Autodesk Fusion 360 part; units mm, degrees
note: some values were not read from the file. Chosen so that the rebuilt part matches the saved one: which bodies a step acts on.
(part 3 of 3)
  arc A266 (-250.9457, 90.0604) -> (-250.4457, 89.5604) centre (-250.4457, 90.0604) ccw
  line L293 (-250.9457, 90.0604) -> (-250.9457, 90.3732)
  line L294 (-250.9457, 90.3732) -> (-252.5563, 90.3732)
  line L295 (-252.5563, 90.3732) -> (-252.5563, 88.75)
  arc A267 (-253.0563, 88.25) -> (-252.5563, 88.75) centre (-253.0563, 88.75) ccw
  line L296 (-253.0563, 88.25) -> (-266.0562, 88.25)
  arc A268 (-266.5562, 88.75) -> (-266.0563, 88.25) centre (-266.0563, 88.75) ccw
  line L297 (-266.5562, 88.75) -> (-266.5562, 90.3732)
  line L298 (-266.5562, 90.3732) -> (-268.1669, 90.3732)
  line L299 (-268.1669, 90.3732) -> (-268.1669, 90.0604)
  arc A269 (-268.6669, 89.5604) -> (-268.1669, 90.0604) centre (-268.6669, 90.0604) ccw
  line L300 (-268.6669, 89.5604) -> (-274.3216, 89.5604)
  arc A270 (-274.8216, 90.0604) -> (-274.3216, 89.5604) centre (-274.3216, 90.0604) ccw
  line L301 (-274.8216, 90.0604) -> (-274.8216, 92.964)
  line L302 (-274.8216, 92.964) -> (-275.1852, 92.964)
  arc A271 (-275.6852, 93.464) -> (-275.1852, 92.964) centre (-275.1852, 93.464) ccw
  line L303 (-275.6852, 93.464) -> (-275.6852, 95.758)
  arc A272 (-83.9875, 88.25) -> (-83.4875, 88.75) centre (-83.9875, 88.75) ccw
  line L304 (-83.9875, 88.25) -> (-96.9875, 88.25)
  arc A273 (-97.4875, 88.75) -> (-96.9875, 88.25) centre (-96.9875, 88.75) ccw
  line L305 (-97.4875, 88.75) -> (-97.4875, 101.75)
  arc A274 (-96.9875, 102.25) -> (-97.4875, 101.75) centre (-96.9875, 101.75) ccw
  line L306 (-96.9875, 102.25) -> (-83.9875, 102.25)
  arc A275 (-83.4875, 101.75) -> (-83.9875, 102.25) centre (-83.9875, 101.75) ccw
  line L307 (-83.4875, 101.75) -> (-83.4875, 88.75)
  arc A276 (-112.5625, 69.2) -> (-112.0625, 69.7) centre (-112.5625, 69.7) ccw
  line L308 (-112.5625, 69.2) -> (-125.5625, 69.2)
  arc A277 (-126.0625, 69.7) -> (-125.5625, 69.2) centre (-125.5625, 69.7) ccw
  line L309 (-126.0625, 69.7) -> (-126.0625, 82.7)
  arc A278 (-125.5625, 83.2) -> (-126.0625, 82.7) centre (-125.5625, 82.7) ccw
  line L310 (-125.5625, 83.2) -> (-112.5625, 83.2)
  arc A279 (-112.0625, 82.7) -> (-112.5625, 83.2) centre (-112.5625, 82.7) ccw
  line L311 (-112.0625, 82.7) -> (-112.0625, 69.7)
  arc A280 (-198.2875, 88.25) -> (-197.7875, 88.75) centre (-198.2875, 88.75) ccw
  line L312 (-198.2875, 88.25) -> (-211.2875, 88.25)
  arc A281 (-211.7875, 88.75) -> (-211.2875, 88.25) centre (-211.2875, 88.75) ccw
  line L313 (-211.7875, 88.75) -> (-211.7875, 101.75)
  arc A282 (-211.2875, 102.25) -> (-211.7875, 101.75) centre (-211.2875, 101.75) ccw
  line L314 (-211.2875, 102.25) -> (-198.2875, 102.25)
  arc A283 (-197.7875, 101.75) -> (-198.2875, 102.25) centre (-198.2875, 101.75) ccw
  line L315 (-197.7875, 101.75) -> (-197.7875, 88.75)
  arc A284 (-207.8125, 69.2) -> (-207.3125, 69.7) centre (-207.8125, 69.7) ccw
  line L316 (-207.8125, 69.2) -> (-220.8125, 69.2)
  arc A285 (-221.3125, 69.7) -> (-220.8125, 69.2) centre (-220.8125, 69.7) ccw
  line L317 (-221.3125, 69.7) -> (-221.3125, 82.7)
  arc A286 (-220.8125, 83.2) -> (-221.3125, 82.7) centre (-220.8125, 82.7) ccw
  line L318 (-220.8125, 83.2) -> (-207.8125, 83.2)
  arc A287 (-207.3125, 82.7) -> (-207.8125, 83.2) centre (-207.8125, 82.7) ccw
  line L319 (-207.3125, 82.7) -> (-207.3125, 69.7)
  arc A288 (-45.8875, 88.25) -> (-45.3875, 88.75) centre (-45.8875, 88.75) ccw
  line L320 (-45.8875, 88.25) -> (-58.8875, 88.25)
  arc A289 (-59.3875, 88.75) -> (-58.8875, 88.25) centre (-58.8875, 88.75) ccw
  line L321 (-59.3875, 88.75) -> (-59.3875, 101.75)
  arc A290 (-58.8875, 102.25) -> (-59.3875, 101.75) centre (-58.8875, 101.75) ccw
  line L322 (-58.8875, 102.25) -> (-45.8875, 102.25)
  arc A291 (-45.3875, 101.75) -> (-45.8875, 102.25) centre (-45.8875, 101.75) ccw
  line L323 (-45.3875, 101.75) -> (-45.3875, 88.75)
  arc A292 (-122.0875, 88.25) -> (-121.5875, 88.75) centre (-122.0875, 88.75) ccw
  line L324 (-122.0875, 88.25) -> (-135.0875, 88.25)
  arc A293 (-135.5875, 88.75) -> (-135.0875, 88.25) centre (-135.0875, 88.75) ccw
  line L325 (-135.5875, 88.75) -> (-135.5875, 101.75)
  arc A294 (-135.0875, 102.25) -> (-135.5875, 101.75) centre (-135.0875, 101.75) ccw
  line L326 (-135.0875, 102.25) -> (-122.0875, 102.25)
  arc A295 (-121.5875, 101.75) -> (-122.0875, 102.25) centre (-122.0875, 101.75) ccw
  line L327 (-121.5875, 101.75) -> (-121.5875, 88.75)
  arc A296 (-179.2375, 88.25) -> (-178.7375, 88.75) centre (-179.2375, 88.75) ccw
  line L328 (-179.2375, 88.25) -> (-192.2375, 88.25)
  arc A297 (-192.7375, 88.75) -> (-192.2375, 88.25) centre (-192.2375, 88.75) ccw
  line L329 (-192.7375, 88.75) -> (-192.7375, 101.75)
  arc A298 (-192.2375, 102.25) -> (-192.7375, 101.75) centre (-192.2375, 101.75) ccw
  line L330 (-192.2375, 102.25) -> (-179.2375, 102.25)
  arc A299 (-178.7375, 101.75) -> (-179.2375, 102.25) centre (-179.2375, 101.75) ccw
  line L331 (-178.7375, 101.75) -> (-178.7375, 88.75)
  arc A300 (-136.375, 31.1) -> (-135.875, 31.6) centre (-136.375, 31.6) ccw
  line L332 (-136.375, 31.1) -> (-149.375, 31.1)
  arc A301 (-149.875, 31.6) -> (-149.375, 31.1) centre (-149.375, 31.6) ccw
  line L333 (-149.875, 31.6) -> (-149.875, 44.6)
  arc A302 (-149.375, 45.1) -> (-149.875, 44.6) centre (-149.375, 44.6) ccw
  line L334 (-149.375, 45.1) -> (-136.375, 45.1)
  arc A303 (-135.875, 44.6) -> (-136.375, 45.1) centre (-136.375, 44.6) ccw
  line L335 (-135.875, 44.6) -> (-135.875, 31.6)
  arc A304 (-93.5125, 69.2) -> (-93.0125, 69.7) centre (-93.5125, 69.7) ccw
  line L336 (-93.5125, 69.2) -> (-106.5125, 69.2)
  arc A305 (-107.0125, 69.7) -> (-106.5125, 69.2) centre (-106.5125, 69.7) ccw
  line L337 (-107.0125, 69.7) -> (-107.0125, 82.7)
  arc A306 (-106.5125, 83.2) -> (-107.0125, 82.7) centre (-106.5125, 82.7) ccw
  line L338 (-106.5125, 83.2) -> (-93.5125, 83.2)
  arc A307 (-93.0125, 82.7) -> (-93.5125, 83.2) centre (-93.5125, 82.7) ccw
  line L339 (-93.0125, 82.7) -> (-93.0125, 69.7)
  arc A308 (-31.6, 50.15) -> (-31.1, 50.65) centre (-31.6, 50.65) ccw
  line L340 (-31.6, 50.15) -> (-44.6, 50.15)
  arc A309 (-45.1, 50.65) -> (-44.6, 50.15) centre (-44.6, 50.65) ccw
  line L341 (-45.1, 50.65) -> (-45.1, 63.65)
  arc A310 (-44.6, 64.15) -> (-45.1, 63.65) centre (-44.6, 63.65) ccw
  line L342 (-44.6, 64.15) -> (-31.6, 64.15)
  arc A311 (-31.1, 63.65) -> (-31.6, 64.15) centre (-31.6, 63.65) ccw
  line L343 (-31.1, 63.65) -> (-31.1, 50.65)
  line L344 (-282.829, 38.608) -> (-282.4654, 38.608)
  arc A312 (-282.4654, 38.608) -> (-281.9654, 39.108) centre (-282.4654, 39.108) ccw
  line L345 (-281.9654, 39.108) -> (-281.9654, 44.204)
  arc A313 (-281.4654, 44.704) -> (-281.9654, 44.204) centre (-281.4654, 44.204) ccw
  line L346 (-281.4654, 44.704) -> (-280.662, 44.704)
  arc A314 (-280.662, 44.704) -> (-280.162, 45.204) centre (-280.662, 45.204) ccw
  line L347 (-280.162, 45.204) -> (-280.162, 45.3724)
  arc A315 (-279.662, 45.8724) -> (-280.162, 45.3724) centre (-279.662, 45.3724) ccw
  line L348 (-279.662, 45.8724) -> (-277.614, 45.8724)
  arc A316 (-277.114, 45.3724) -> (-277.614, 45.8724) centre (-277.614, 45.3724) ccw
  line L349 (-277.114, 45.3724) -> (-277.114, 45.204)
  arc A317 (-277.114, 45.204) -> (-276.614, 44.704) centre (-276.614, 45.204) ccw
  line L350 (-276.614, 44.704) -> (-275.3106, 44.704)
  line L351 (-275.3106, 44.704) -> (-275.3106, 44.4166)
  arc A318 (-275.3106, 44.4166) -> (-274.8106, 43.9166) centre (-274.8106, 44.4166) ccw
  line L352 (-274.8106, 43.9166) -> (-273.7, 43.9166)
  line L353 (-273.7, 43.9166) -> (-273.7, 44.6)
  arc A319 (-273.2, 45.1) -> (-273.7, 44.6) centre (-273.2, 44.6) ccw
  line L354 (-273.2, 45.1) -> (-260.2, 45.1)
  arc A320 (-259.7, 44.6) -> (-260.2, 45.1) centre (-260.2, 44.6) ccw
  line L355 (-259.7, 44.6) -> (-259.7, 43.9166)
  line L356 (-259.7, 43.9166) -> (-258.5894, 43.9166)
  arc A321 (-258.5894, 43.9166) -> (-258.0894, 44.4166) centre (-258.5894, 44.4166) ccw
  line L357 (-258.0894, 44.4166) -> (-258.0894, 44.704)
  line L358 (-258.0894, 44.704) -> (-256.786, 44.704)
  arc A322 (-256.786, 44.704) -> (-256.286, 45.204) centre (-256.786, 45.204) ccw
  line L359 (-256.286, 45.204) -> (-256.286, 45.3724)
  arc A323 (-255.786, 45.8724) -> (-256.286, 45.3724) centre (-255.786, 45.3724) ccw
  line L360 (-255.786, 45.8724) -> (-253.738, 45.8724)
  arc A324 (-253.238, 45.3724) -> (-253.738, 45.8724) centre (-253.738, 45.3724) ccw
  line L361 (-253.238, 45.3724) -> (-253.238, 45.204)
  arc A325 (-253.238, 45.204) -> (-252.738, 44.704) centre (-252.738, 45.204) ccw
  line L362 (-252.738, 44.704) -> (-251.9346, 44.704)
  arc A326 (-251.4346, 44.204) -> (-251.9346, 44.704) centre (-251.9346, 44.204) ccw
  line L363 (-251.4346, 44.204) -> (-251.4346, 39.108)
  arc A327 (-251.4346, 39.108) -> (-250.9346, 38.608) centre (-250.9346, 39.108) ccw
  line L364 (-250.9346, 38.608) -> (-250.571, 38.608)
  line L365 (-250.571, 38.608) -> (-250.571, 36.314)
  arc A328 (-251.071, 35.814) -> (-250.571, 36.314) centre (-251.071, 36.314) ccw
  line L366 (-251.071, 35.814) -> (-251.4346, 35.814)
  line L367 (-251.4346, 35.814) -> (-251.4346, 32.9104)
  arc A329 (-251.9346, 32.4104) -> (-251.4346, 32.9104) centre (-251.9346, 32.9104) ccw
  line L368 (-251.9346, 32.4104) -> (-257.5894, 32.4104)
  arc A330 (-258.0894, 32.9104) -> (-257.5894, 32.4104) centre (-257.5894, 32.9104) ccw
  line L369 (-258.0894, 32.9104) -> (-258.0894, 33.2232)
  line L370 (-258.0894, 33.2232) -> (-259.7, 33.2232)
  line L371 (-259.7, 33.2232) -> (-259.7, 31.6)
  arc A331 (-260.2, 31.1) -> (-259.7, 31.6) centre (-260.2, 31.6) ccw
  line L372 (-260.2, 31.1) -> (-273.2, 31.1)
  arc A332 (-273.7, 31.6) -> (-273.2, 31.1) centre (-273.2, 31.6) ccw
  line L373 (-273.7, 31.6) -> (-273.7, 33.2232)
  line L374 (-273.7, 33.2232) -> (-275.3106, 33.2232)
  line L375 (-275.3106, 33.2232) -> (-275.3106, 32.9104)
  arc A333 (-275.8106, 32.4104) -> (-275.3106, 32.9104) centre (-275.8106, 32.9104) ccw
  line L376 (-275.8106, 32.4104) -> (-281.4654, 32.4104)
  arc A334 (-281.9654, 32.9104) -> (-281.4654, 32.4104) centre (-281.4654, 32.9104) ccw
  line L377 (-281.9654, 32.9104) -> (-281.9654, 35.814)
  line L378 (-281.9654, 35.814) -> (-282.329, 35.814)
  arc A335 (-282.829, 36.314) -> (-282.329, 35.814) centre (-282.329, 36.314) ccw
  line L379 (-282.829, 36.314) -> (-282.829, 38.608)
  arc A336 (-50.65, 50.15) -> (-50.15, 50.65) centre (-50.65, 50.65) ccw
  line L380 (-50.65, 50.15) -> (-63.65, 50.15)
  arc A337 (-64.15, 50.65) -> (-63.65, 50.15) centre (-63.65, 50.65) ccw
  line L381 (-64.15, 50.65) -> (-64.15, 63.65)
  arc A338 (-63.65, 64.15) -> (-64.15, 63.65) centre (-63.65, 63.65) ccw
  line L382 (-63.65, 64.15) -> (-50.65, 64.15)
  arc A339 (-50.15, 63.65) -> (-50.65, 64.15) centre (-50.65, 63.65) ccw
  line L383 (-50.15, 63.65) -> (-50.15, 50.65)
  arc A340 (-3.025, 2.525) -> (-2.525, 3.025) centre (-3.025, 3.025) ccw
  line L384 (-3.025, 2.525) -> (-16.025, 2.525)
  arc A341 (-16.525, 3.025) -> (-16.025, 2.525) centre (-16.025, 3.025) ccw
  line L385 (-16.525, 3.025) -> (-16.525, 16.025)
  arc A342 (-16.025, 16.525) -> (-16.525, 16.025) centre (-16.025, 16.025) ccw
  line L386 (-16.025, 16.525) -> (-3.025, 16.525)
  arc A343 (-2.525, 16.025) -> (-3.025, 16.525) centre (-3.025, 16.025) ccw
  line L387 (-2.525, 16.025) -> (-2.525, 3.025)
  arc A344 (-88.75, 50.15) -> (-88.25, 50.65) centre (-88.75, 50.65) ccw
  line L388 (-88.75, 50.15) -> (-101.75, 50.15)
  arc A345 (-102.25, 50.65) -> (-101.75, 50.15) centre (-101.75, 50.65) ccw
  line L389 (-102.25, 50.65) -> (-102.25, 63.65)
  arc A346 (-101.75, 64.15) -> (-102.25, 63.65) centre (-101.75, 63.65) ccw
  line L390 (-101.75, 64.15) -> (-88.75, 64.15)
  arc A347 (-88.25, 63.65) -> (-88.75, 64.15) centre (-88.75, 63.65) ccw
  line L391 (-88.25, 63.65) -> (-88.25, 50.65)
  arc A348 (-145.9, 50.15) -> (-145.4, 50.65) centre (-145.9, 50.65) ccw
  line L392 (-145.9, 50.15) -> (-158.9, 50.15)
  arc A349 (-159.4, 50.65) -> (-158.9, 50.15) centre (-158.9, 50.65) ccw
  line L393 (-159.4, 50.65) -> (-159.4, 63.65)
  arc A350 (-158.9, 64.15) -> (-159.4, 63.65) centre (-158.9, 63.65) ccw
  line L394 (-158.9, 64.15) -> (-145.9, 64.15)
  arc A351 (-145.4, 63.65) -> (-145.9, 64.15) centre (-145.9, 63.65) ccw
  line L395 (-145.4, 63.65) -> (-145.4, 50.65)
  arc A352 (-60.175, 2.525) -> (-59.675, 3.025) centre (-60.175, 3.025) ccw
  line L396 (-60.175, 2.525) -> (-73.175, 2.525)
  arc A353 (-73.675, 3.025) -> (-73.175, 2.525) centre (-73.175, 3.025) ccw
  line L397 (-73.675, 3.025) -> (-73.675, 16.025)
  arc A354 (-73.175, 16.525) -> (-73.675, 16.025) centre (-73.175, 16.025) ccw
  line L398 (-73.175, 16.525) -> (-60.175, 16.525)
  arc A355 (-59.675, 16.025) -> (-60.175, 16.525) centre (-60.175, 16.025) ccw
  line L399 (-59.675, 16.025) -> (-59.675, 3.025)
  arc A356 (-293.5375, 31.1) -> (-293.0375, 31.6) centre (-293.5375, 31.6) ccw
  line L400 (-293.5375, 31.1) -> (-306.5375, 31.1)
  arc A357 (-307.0375, 31.6) -> (-306.5375, 31.1) centre (-306.5375, 31.6) ccw
  line L401 (-307.0375, 31.6) -> (-307.0375, 44.6)
  arc A358 (-306.5375, 45.1) -> (-307.0375, 44.6) centre (-306.5375, 44.6) ccw
  line L402 (-306.5375, 45.1) -> (-293.5375, 45.1)
  arc A359 (-293.0375, 44.6) -> (-293.5375, 45.1) centre (-293.5375, 44.6) ccw
  line L403 (-293.0375, 44.6) -> (-293.0375, 31.6)
  arc A360 (-312.5875, 2.525) -> (-312.0875, 3.025) centre (-312.5875, 3.025) ccw
  line L404 (-312.5875, 2.525) -> (-325.5875, 2.525)
  arc A361 (-326.0875, 3.025) -> (-325.5875, 2.525) centre (-325.5875, 3.025) ccw
  line L405 (-326.0875, 3.025) -> (-326.0875, 16.025)
  arc A362 (-325.5875, 16.525) -> (-326.0875, 16.025) centre (-325.5875, 16.025) ccw
  line L406 (-325.5875, 16.525) -> (-312.5875, 16.525)
  arc A363 (-312.0875, 16.025) -> (-312.5875, 16.525) centre (-312.5875, 16.025) ccw
  line L407 (-312.0875, 16.025) -> (-312.0875, 3.025)
  arc A364 (-164.95, 50.15) -> (-164.45, 50.65) centre (-164.95, 50.65) ccw
  line L408 (-164.95, 50.15) -> (-177.95, 50.15)
  arc A365 (-178.45, 50.65) -> (-177.95, 50.15) centre (-177.95, 50.65) ccw
  line L409 (-178.45, 50.65) -> (-178.45, 63.65)
  arc A366 (-177.95, 64.15) -> (-178.45, 63.65) centre (-177.95, 63.65) ccw
  line L410 (-177.95, 64.15) -> (-164.95, 64.15)
  arc A367 (-164.45, 63.65) -> (-164.95, 64.15) centre (-164.95, 63.65) ccw
  line L411 (-164.45, 63.65) -> (-164.45, 50.65)
  arc A368 (-107.8, 50.15) -> (-107.3, 50.65) centre (-107.8, 50.65) ccw
  line L412 (-107.8, 50.15) -> (-120.8, 50.15)
  arc A369 (-121.3, 50.65) -> (-120.8, 50.15) centre (-120.8, 50.65) ccw
  line L413 (-121.3, 50.65) -> (-121.3, 63.65)
  arc A370 (-120.8, 64.15) -> (-121.3, 63.65) centre (-120.8, 63.65) ccw
  line L414 (-120.8, 64.15) -> (-107.8, 64.15)
  arc A371 (-107.3, 63.65) -> (-107.8, 64.15) centre (-107.8, 63.65) ccw
  line L415 (-107.3, 63.65) -> (-107.3, 50.65)
  arc A372 (-150.6625, 69.2) -> (-150.1625, 69.7) centre (-150.6625, 69.7) ccw
  line L416 (-150.6625, 69.2) -> (-163.6625, 69.2)
  arc A373 (-164.1625, 69.7) -> (-163.6625, 69.2) centre (-163.6625, 69.7) ccw
  line L417 (-164.1625, 69.7) -> (-164.1625, 82.7)
  arc A374 (-163.6625, 83.2) -> (-164.1625, 82.7) centre (-163.6625, 82.7) ccw
  line L418 (-163.6625, 83.2) -> (-150.6625, 83.2)
  arc A375 (-150.1625, 82.7) -> (-150.6625, 83.2) centre (-150.6625, 82.7) ccw
  line L419 (-150.1625, 82.7) -> (-150.1625, 69.7)
  arc A376 (-174.475, 31.1) -> (-173.975, 31.6) centre (-174.475, 31.6) ccw
  line L420 (-174.475, 31.1) -> (-187.475, 31.1)
  arc A377 (-187.975, 31.6) -> (-187.475, 31.1) centre (-187.475, 31.6) ccw
  line L421 (-187.975, 31.6) -> (-187.975, 44.6)
  arc A378 (-187.475, 45.1) -> (-187.975, 44.6) centre (-187.475, 44.6) ccw
  line L422 (-187.475, 45.1) -> (-174.475, 45.1)
  arc A379 (-173.975, 44.6) -> (-174.475, 45.1) centre (-174.475, 44.6) ccw
  line L423 (-173.975, 44.6) -> (-173.975, 31.6)
  arc A380 (-241.15, 50.15) -> (-240.65, 50.65) centre (-241.15, 50.65) ccw
  line L424 (-241.15, 50.15) -> (-254.15, 50.15)
  arc A381 (-254.65, 50.65) -> (-254.15, 50.15) centre (-254.15, 50.65) ccw
  line L425 (-254.65, 50.65) -> (-254.65, 63.65)
  arc A382 (-254.15, 64.15) -> (-254.65, 63.65) centre (-254.15, 63.65) ccw
  line L426 (-254.15, 64.15) -> (-241.15, 64.15)
  arc A383 (-240.65, 63.65) -> (-241.15, 64.15) centre (-241.15, 63.65) ccw
  line L427 (-240.65, 63.65) -> (-240.65, 50.65)
  arc A384 (-5.4063, 88.25) -> (-4.9063, 88.75) centre (-5.4062, 88.75) ccw
  line L428 (-5.4062, 88.25) -> (-18.4062, 88.25)
  arc A385 (-18.9062, 88.75) -> (-18.4062, 88.25) centre (-18.4062, 88.75) ccw
  line L429 (-18.9062, 88.75) -> (-18.9062, 101.75)
  arc A386 (-18.4062, 102.25) -> (-18.9063, 101.75) centre (-18.4063, 101.75) ccw
  line L430 (-18.4062, 102.25) -> (-5.4062, 102.25)
  arc A387 (-4.9062, 101.75) -> (-5.4062, 102.25) centre (-5.4062, 101.75) ccw
  line L431 (-4.9062, 101.75) -> (-4.9063, 88.75)
  arc A388 (-10.1687, 69.2) -> (-9.6687, 69.7) centre (-10.1687, 69.7) ccw
  line L432 (-10.1687, 69.2) -> (-23.1687, 69.2)
  arc A389 (-23.6687, 69.7) -> (-23.1687, 69.2) centre (-23.1688, 69.7) ccw
  line L433 (-23.6687, 69.7) -> (-23.6688, 82.7)
  arc A390 (-23.1687, 83.2) -> (-23.6687, 82.7) centre (-23.1688, 82.7) ccw
  line L434 (-23.1687, 83.2) -> (-10.1687, 83.2)
  arc A391 (-9.6687, 82.7) -> (-10.1687, 83.2) centre (-10.1688, 82.7) ccw
  line L435 (-9.6687, 82.7) -> (-9.6687, 69.7)
  arc A392 (-36.3625, 69.2) -> (-35.8625, 69.7) centre (-36.3625, 69.7) ccw
  line L436 (-36.3625, 69.2) -> (-49.3625, 69.2)
  arc A393 (-49.8625, 69.7) -> (-49.3625, 69.2) centre (-49.3625, 69.7) ccw
  line L437 (-49.8625, 69.7) -> (-49.8625, 82.7)
  arc A394 (-49.3625, 83.2) -> (-49.8625, 82.7) centre (-49.3625, 82.7) ccw
  line L438 (-49.3625, 83.2) -> (-36.3625, 83.2)
  arc A395 (-35.8625, 82.7) -> (-36.3625, 83.2) centre (-36.3625, 82.7) ccw
  line L439 (-35.8625, 82.7) -> (-35.8625, 69.7)
  arc A396 (-7.7875, 50.15) -> (-7.2875, 50.65) centre (-7.7875, 50.65) ccw
  line L440 (-7.7875, 50.15) -> (-20.7875, 50.15)
  arc A397 (-21.2875, 50.65) -> (-20.7875, 50.15) centre (-20.7875, 50.65) ccw
  line L441 (-21.2875, 50.65) -> (-21.2875, 63.65)
  arc A398 (-20.7875, 64.15) -> (-21.2875, 63.65) centre (-20.7875, 63.65) ccw
  line L442 (-20.7875, 64.15) -> (-7.7875, 64.15)
  arc A399 (-7.2875, 63.65) -> (-7.7875, 64.15) centre (-7.7875, 63.65) ccw
  line L443 (-7.2875, 63.65) -> (-7.2875, 50.65)
  arc A400 (-331.6375, 50.15) -> (-331.1375, 50.65) centre (-331.6375, 50.65) ccw
  line L444 (-331.6375, 50.15) -> (-344.6375, 50.15)
  arc A401 (-345.1375, 50.65) -> (-344.6375, 50.15) centre (-344.6375, 50.65) ccw
  line L445 (-345.1375, 50.65) -> (-345.1375, 63.65)
  arc A402 (-344.6375, 64.15) -> (-345.1375, 63.65) centre (-344.6375, 63.65) ccw
  line L446 (-344.6375, 64.15) -> (-331.6375, 64.15)
  arc A403 (-331.1375, 63.65) -> (-331.6375, 64.15) centre (-331.6375, 63.65) ccw
  line L447 (-331.1375, 63.65) -> (-331.1375, 50.65)
  arc A404 (-41.125, 2.525) -> (-40.625, 3.025) centre (-41.125, 3.025) ccw
  line L448 (-41.125, 2.525) -> (-54.125, 2.525)
  arc A405 (-54.625, 3.025) -> (-54.125, 2.525) centre (-54.125, 3.025) ccw
  line L449 (-54.625, 3.025) -> (-54.625, 16.025)
  arc A406 (-54.125, 16.525) -> (-54.625, 16.025) centre (-54.125, 16.025) ccw
  line L450 (-54.125, 16.525) -> (-41.125, 16.525)
  arc A407 (-40.625, 16.025) -> (-41.125, 16.525) centre (-41.125, 16.025) ccw
  line L451 (-40.625, 16.025) -> (-40.625, 3.025)
  arc A408 (-293.5375, 50.15) -> (-293.0375, 50.65) centre (-293.5375, 50.65) ccw
  line L452 (-293.5375, 50.15) -> (-306.5375, 50.15)
  arc A409 (-307.0375, 50.65) -> (-306.5375, 50.15) centre (-306.5375, 50.65) ccw
  line L453 (-307.0375, 50.65) -> (-307.0375, 63.65)
  arc A410 (-306.5375, 64.15) -> (-307.0375, 63.65) centre (-306.5375, 63.65) ccw
  line L454 (-306.5375, 64.15) -> (-293.5375, 64.15)
  arc A411 (-293.0375, 63.65) -> (-293.5375, 64.15) centre (-293.5375, 63.65) ccw
  line L455 (-293.0375, 63.65) -> (-293.0375, 50.65)
  arc A412 (-226.8625, 69.2) -> (-226.3625, 69.7) centre (-226.8625, 69.7) ccw
  line L456 (-226.8625, 69.2) -> (-239.8625, 69.2)
  arc A413 (-240.3625, 69.7) -> (-239.8625, 69.2) centre (-239.8625, 69.7) ccw
  line L457 (-240.3625, 69.7) -> (-240.3625, 82.7)
  arc A414 (-239.8625, 83.2) -> (-240.3625, 82.7) centre (-239.8625, 82.7) ccw
  line L458 (-239.8625, 83.2) -> (-226.8625, 83.2)
  arc A415 (-226.3625, 82.7) -> (-226.8625, 83.2) centre (-226.8625, 82.7) ccw
  line L459 (-226.3625, 82.7) -> (-226.3625, 69.7)
  arc A416 (-222.1, 50.15) -> (-221.6, 50.65) centre (-222.1, 50.65) ccw
  line L460 (-222.1, 50.15) -> (-235.1, 50.15)
  arc A417 (-235.6, 50.65) -> (-235.1, 50.15) centre (-235.1, 50.65) ccw
  line L461 (-235.6, 50.65) -> (-235.6, 63.65)
  arc A418 (-235.1, 64.15) -> (-235.6, 63.65) centre (-235.1, 63.65) ccw
  line L462 (-235.1, 64.15) -> (-222.1, 64.15)
  arc A419 (-221.6, 63.65) -> (-222.1, 64.15) centre (-222.1, 63.65) ccw
  line L463 (-221.6, 63.65) -> (-221.6, 50.65)
  arc A420 (-69.7, 50.15) -> (-69.2, 50.65) centre (-69.7, 50.65) ccw
  line L464 (-69.7, 50.15) -> (-82.7, 50.15)
  arc A421 (-83.2, 50.65) -> (-82.7, 50.15) centre (-82.7, 50.65) ccw
  line L465 (-83.2, 50.65) -> (-83.2, 63.65)
  arc A422 (-82.7, 64.15) -> (-83.2, 63.65) centre (-82.7, 63.65) ccw
  line L466 (-82.7, 64.15) -> (-69.7, 64.15)
  arc A423 (-69.2, 63.65) -> (-69.7, 64.15) centre (-69.7, 63.65) ccw
  line L467 (-69.2, 63.65) -> (-69.2, 50.65)
  arc A424 (-293.5375, 69.2) -> (-293.0375, 69.7) centre (-293.5375, 69.7) ccw
  line L468 (-293.5375, 69.2) -> (-306.5375, 69.2)
  arc A425 (-307.0375, 69.7) -> (-306.5375, 69.2) centre (-306.5375, 69.7) ccw
  line L469 (-307.0375, 69.7) -> (-307.0375, 82.7)
  arc A426 (-306.5375, 83.2) -> (-307.0375, 82.7) centre (-306.5375, 82.7) ccw
  line L470 (-306.5375, 83.2) -> (-293.5375, 83.2)
  arc A427 (-293.0375, 82.7) -> (-293.5375, 83.2) centre (-293.5375, 82.7) ccw
  line L471 (-293.0375, 82.7) -> (-293.0375, 69.7)
  arc A428 (-293.5375, 2.525) -> (-293.0375, 3.025) centre (-293.5375, 3.025) ccw
  line L472 (-293.5375, 2.525) -> (-306.5375, 2.525)
  arc A429 (-307.0375, 3.025) -> (-306.5375, 2.525) centre (-306.5375, 3.025) ccw
  line L473 (-307.0375, 3.025) -> (-307.0375, 16.025)
  arc A430 (-306.5375, 16.525) -> (-307.0375, 16.025) centre (-306.5375, 16.025) ccw
  line L474 (-306.5375, 16.525) -> (-293.5375, 16.525)
  arc A431 (-293.0375, 16.025) -> (-293.5375, 16.525) centre (-293.5375, 16.025) ccw
  line L475 (-293.0375, 16.025) -> (-293.0375, 3.025)
  arc A432 (-203.05, 50.15) -> (-202.55, 50.65) centre (-203.05, 50.65) ccw
  line L476 (-203.05, 50.15) -> (-216.05, 50.15)
  arc A433 (-216.55, 50.65) -> (-216.05, 50.15) centre (-216.05, 50.65) ccw
  line L477 (-216.55, 50.65) -> (-216.55, 63.65)
  arc A434 (-216.05, 64.15) -> (-216.55, 63.65) centre (-216.05, 63.65) ccw
  line L478 (-216.05, 64.15) -> (-203.05, 64.15)
  arc A435 (-202.55, 63.65) -> (-203.05, 64.15) centre (-203.05, 63.65) ccw
  line L479 (-202.55, 63.65) -> (-202.55, 50.65)
  arc A436 (-55.4125, 69.2) -> (-54.9125, 69.7) centre (-55.4125, 69.7) ccw
  line L480 (-55.4125, 69.2) -> (-68.4125, 69.2)
  arc A437 (-68.9125, 69.7) -> (-68.4125, 69.2) centre (-68.4125, 69.7) ccw
  line L481 (-68.9125, 69.7) -> (-68.9125, 82.7)
  arc A438 (-68.4125, 83.2) -> (-68.9125, 82.7) centre (-68.4125, 82.7) ccw
  line L482 (-68.4125, 83.2) -> (-55.4125, 83.2)
  arc A439 (-54.9125, 82.7) -> (-55.4125, 83.2) centre (-55.4125, 82.7) ccw
  line L483 (-54.9125, 82.7) -> (-54.9125, 69.7)
  arc A440 (-26.8375, 88.25) -> (-26.3375, 88.75) centre (-26.8375, 88.75) ccw
  line L484 (-26.8375, 88.25) -> (-39.8375, 88.25)
  arc A441 (-40.3375, 88.75) -> (-39.8375, 88.25) centre (-39.8375, 88.75) ccw
  line L485 (-40.3375, 88.75) -> (-40.3375, 101.75)
  arc A442 (-39.8375, 102.25) -> (-40.3375, 101.75) centre (-39.8375, 101.75) ccw
  line L486 (-39.8375, 102.25) -> (-26.8375, 102.25)
  arc A443 (-26.3375, 101.75) -> (-26.8375, 102.25) centre (-26.8375, 101.75) ccw
  line L487 (-26.3375, 101.75) -> (-26.3375, 88.75)
  arc A444 (-312.5875, 31.1) -> (-312.0875, 31.6) centre (-312.5875, 31.6) ccw
  line L488 (-312.5875, 31.1) -> (-325.5875, 31.1)
  arc A445 (-326.0875, 31.6) -> (-325.5875, 31.1) centre (-325.5875, 31.6) ccw
  line L489 (-326.0875, 31.6) -> (-326.0875, 44.6)
  arc A446 (-325.5875, 45.1) -> (-326.0875, 44.6) centre (-325.5875, 44.6) ccw
  line L490 (-325.5875, 45.1) -> (-312.5875, 45.1)
  arc A447 (-312.0875, 44.6) -> (-312.5875, 45.1) centre (-312.5875, 44.6) ccw
  line L491 (-312.0875, 44.6) -> (-312.0875, 31.6)
  arc A448 (-231.625, 2.525) -> (-231.125, 3.025) centre (-231.625, 3.025) ccw
  line L492 (-231.625, 2.525) -> (-244.625, 2.525)
  arc A449 (-245.125, 3.025) -> (-244.625, 2.525) centre (-244.625, 3.025) ccw
  line L493 (-245.125, 3.025) -> (-245.125, 16.025)
  arc A450 (-244.625, 16.525) -> (-245.125, 16.025) centre (-244.625, 16.025) ccw
  line L494 (-244.625, 16.525) -> (-231.625, 16.525)
  arc A451 (-231.125, 16.025) -> (-231.625, 16.525) centre (-231.625, 16.025) ccw
  line L495 (-231.125, 16.025) -> (-231.125, 3.025)
  arc A452 (-312.5875, 50.15) -> (-312.0875, 50.65) centre (-312.5875, 50.65) ccw
  line L496 (-312.5875, 50.15) -> (-325.5875, 50.15)
  arc A453 (-326.0875, 50.65) -> (-325.5875, 50.15) centre (-325.5875, 50.65) ccw
  line L497 (-326.0875, 50.65) -> (-326.0875, 63.65)
  arc A454 (-325.5875, 64.15) -> (-326.0875, 63.65) centre (-325.5875, 63.65) ccw
  line L498 (-325.5875, 64.15) -> (-312.5875, 64.15)
  arc A455 (-312.0875, 63.65) -> (-312.5875, 64.15) centre (-312.5875, 63.65) ccw
  line L499 (-312.0875, 63.65) -> (-312.0875, 50.65)
  line L500 (2, -3) -> (2, 128.825)
  line L501 (2, 128.825) -> (-379.1625, 128.825)
  line L502 (-379.1625, 128.825) -> (-379.1625, -3)
  line L503 (-379.1625, -3) -> (2, -3)
  line L504 (2, 62.9125) -> (-379.1625, 62.9125)
  line L505 (-188.5813, 62.9125) -> (-188.5813, -3)
  line L506 (-188.5813, 62.9125) -> (-188.5813, 128.825)
  constraint midpoint L500 L504.start
  constraint midpoint L502 L504.end
  constraint midpoint L504 L505.start
  constraint midpoint L503 L505.end
  constraint midpoint L501 L506.end
split "Split1" by curves path "Sketch2" along L506 L505 bodies 1 makes body 2 at (367.8208, 0, 63.1583)
move_body "Move1" bodies 2 to x (1, 0, 0) y (0, 1, 0) z (0, 0, 1) at (-190.0062, 0, 133.5727)
